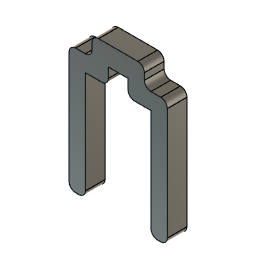
Hook holder small v6 (Autodesk Fusion 360 design; units mm, degrees)
Autodesk Fusion 360 part; units mm, degrees
note: some values were not read from the file. Chosen so that the rebuilt part matches the saved one: which bodies a step acts on. Set by a fixed rule: which face or edge a step refers to.
sketch "Sketch1" plane through (0, 0, 0) normal (0, 0, 1) x (1, 0, 0)
  line L0 (10, 10) -> (15, 10)
  line L1 (15, 10) -> (15, 4)
  line L2 (15, 4) -> (10, 4)
  line L3 (10, 4) -> (10, 10)
  line L4 (10, 7) -> (-20, 7) construction
  line L5 (-20, 10) -> (-15, 10)
  line L6 (-15, 10) -> (-15, 4)
  line L7 (-15, 4) -> (-20, 4)
  line L8 (-20, 4) -> (-20, 10)
  dimension "d1" = 5
  dimension "d2" = 6
  dimension "d3" = 30
  dimension "d4" = 5
  dimension "d5" = 6
  constraint horizontal L0
  constraint vertical L1
  constraint horizontal L2
  constraint vertical L3
  constraint midpoint L3 L4.start
  constraint perpendicular L3 L4
  constraint horizontal L5
  constraint vertical L6
  constraint horizontal L7
  constraint vertical L8
  measures "d1" distance of L0.start L0.end
  measures "d2" distance of L0.start L2.end
  measures "d3" distance of L4.start L4.end
  measures "d4" distance of L5.start L5.end
  measures "d5" distance of L5.start L7.end
extrude "Extrude1" add sketch "Sketch1" along normal blind 34.231 makes body 1 at (-15, 8, 11.4103) makes body 2 at (15, 8, 11.4103)
sketch "Sketch2" plane through (-15, 0, 0) normal (1, 0, 0) x (0, 1, 0)
  line L0 (4, 0) -> (10, 0)
  line L1 (10, 0) -> (10, 34.231)
  line L2 (10, 34.231) -> (4, 34.231)
  line L3 (4, 34.231) -> (4, 0)
  line L4 (4, 34.231) -> (10, 34.231)
  line L5 (10, 34.231) -> (10, 29.231)
  line L6 (10, 29.231) -> (4, 29.231)
  line L7 (4, 29.231) -> (4, 34.231)
  dimension "d8" = 5
  constraint horizontal L4
  constraint vertical L5
  constraint horizontal L6
  constraint vertical L7
  constraint coincident L2.end L3.start
  measures "d8" distance of L2.end L6.end
extrude "Extrude2" add sketch "Sketch2" along normal blind 20 contours L1 L2 L3 L4 L5 L6 L7 bodies 1
move_body "Move1" bodies 2 to x (1, 0, 0) y (0, 1, 0) z (0, 0, 1) at (-5, 0, 0)
combine "Combine1" operation add target body 1 tool bodies 2
sketch "Sketch3" plane through (0, 0, 34.231) normal (0, 0, 1) x (-1, 0, 0)
  line L0 (20, -4) -> (-10, -4)
  line L1 (-10, -4) -> (-10, -10)
  line L2 (-10, -10) -> (20, -10)
  line L3 (20, -10) -> (20, -4)
  line L4 (-10, -10) -> (2, -10)
  line L5 (2, -10) -> (2, -4)
  line L6 (2, -4) -> (-10, -4)
  line L7 (-10, -4) -> (-10, -10)
  line L8 (20, -10) -> (8, -10)
  line L9 (8, -10) -> (8, -4)
  line L10 (8, -4) -> (20, -4)
  line L11 (20, -4) -> (20, -10)
  line L12 (2, -10) -> (-3, -10)
  line L13 (-3, -10) -> (-3, -4)
  line L14 (-3, -4) -> (2, -4)
  line L15 (2, -4) -> (2, -10)
  line L16 (8, -10) -> (13, -10)
  line L17 (13, -10) -> (13, -4)
  line L18 (13, -4) -> (8, -4)
  line L19 (8, -4) -> (8, -10)
  constraint horizontal L4
  constraint vertical L5
  constraint horizontal L6
  constraint vertical L7
  constraint coincident L0 L5.end
  constraint coincident L1.end L2.start
  constraint horizontal L8
  constraint vertical L9
  constraint horizontal L10
  constraint vertical L11
  constraint coincident L0 L9.end
  constraint coincident L2.end L3.start
  constraint horizontal L12
  constraint vertical L13
  constraint horizontal L14
  constraint vertical L15
  constraint coincident L6 L13.end
  constraint horizontal L16
  constraint vertical L17
  constraint horizontal L18
  constraint vertical L19
  constraint coincident L10 L17.end
extrude "Extrude3" add sketch "Sketch3" along normal blind 6 contours L0 L2 L8 L9 L10 L16 L17 L18 L19 | L0 L2 L4 L5 L6 L12 L13 L14 L15 bodies 1
extrude "Extrude4" cut 1 faces at (-6, 8, 34.231) along direction (0, 0, -1) blind 5 on bodies 1 bodies 1 makes body 3 at (10, 8, 11.4103)
sketch "Sketch4" plane through (-8, 0, 0) normal (1, 0, 0) x (0, 1, 0)
  line L0 (10, 29.231) -> (10, 40.231)
  line L1 (10, 40.231) -> (4, 40.231)
  line L2 (4, 40.231) -> (4, 29.231)
  line L3 (4, 29.231) -> (10, 29.231)
  line L4 (4, 40.231) -> (10, 40.231)
  line L5 (10, 40.231) -> (10, 34.231)
  line L6 (10, 34.231) -> (4, 34.231)
  line L7 (4, 34.231) -> (4, 40.231)
  dimension "d15" = 6
  constraint horizontal L4
  constraint vertical L5
  constraint horizontal L6
  constraint vertical L7
  constraint coincident L0 L5.end
  constraint coincident L1.end L2.start
  measures "d15" distance of L1.end L6.end
extrude "Extrude5" add sketch "Sketch4" along normal blind 6 contours L0 L1 L2 L4 L5 L6 L7 bodies 1 3
fillet "Fillet1" radius 2 8 edges at (3, 7, 40.231) (3, 7, 34.231) (10, 7, 34.231) (-13, 7, 40.231) (-13, 7, 34.231) (-20, 7, 34.231) (-8, 7, 29.231) (-2, 7, 29.231) on bodies 1
extrude "Extrude6" add 2 faces at (-18.3333, 8, 0) (6.6667, 8, 0) along direction (0, 0, -1) blind 4 on bodies 1 bodies 1
fillet "Fillet2" radius 2 4 edges at (-15, 7, -4) (-20, 7, -4) (5, 7, -4) (10, 7, -4) on bodies 1
sketch "Sketch6" plane through (0, 4, 0) normal (0, -1, 0) x (1, 0, 0)
  arc A0 (8, -4) -> (10, -2) centre (8, -2) ccw
  line L0 (10, -2) -> (10, 32.231)
  arc A1 (10, 32.231) -> (8, 34.231) centre (8, 32.231) ccw
  line L1 (8, 34.231) -> (5, 34.231)
  arc A2 (3, 36.231) -> (5, 34.231) centre (5, 36.231) ccw
  line L2 (3, 36.231) -> (3, 38.231)
  arc A3 (3, 38.231) -> (1, 40.231) centre (1, 38.231) ccw
  line L3 (1, 40.231) -> (-11, 40.231)
  arc A4 (-11, 40.231) -> (-13, 38.231) centre (-11, 38.231) ccw
  line L4 (-13, 38.231) -> (-13, 36.231)
  arc A5 (-15, 34.231) -> (-13, 36.231) centre (-15, 36.231) ccw
  line L5 (-15, 34.231) -> (-18, 34.231)
  arc A6 (-18, 34.231) -> (-20, 32.231) centre (-18, 32.231) ccw
  line L6 (-20, 32.231) -> (-20, -2)
  arc A7 (-20, -2) -> (-18, -4) centre (-18, -2) ccw
  line L7 (-18, -4) -> (-17, -4)
  arc A8 (-17, -4) -> (-15, -2) centre (-17, -2) ccw
  line L8 (-15, -2) -> (-15, 29.231)
  line L9 (-15, 29.231) -> (-10, 29.231)
  arc A9 (-10, 29.231) -> (-8, 31.231) centre (-10, 31.231) ccw
  line L10 (-8, 31.231) -> (-8, 34.231)
  line L11 (-8, 34.231) -> (-2, 34.231)
  line L12 (-2, 34.231) -> (-2, 31.231)
  arc A10 (-2, 31.231) -> (0, 29.231) centre (0, 31.231) ccw
  line L13 (0, 29.231) -> (5, 29.231)
  line L14 (5, 29.231) -> (5, -2)
  arc A11 (5, -2) -> (7, -4) centre (7, -2) ccw
  line L15 (7, -4) -> (8, -4)
